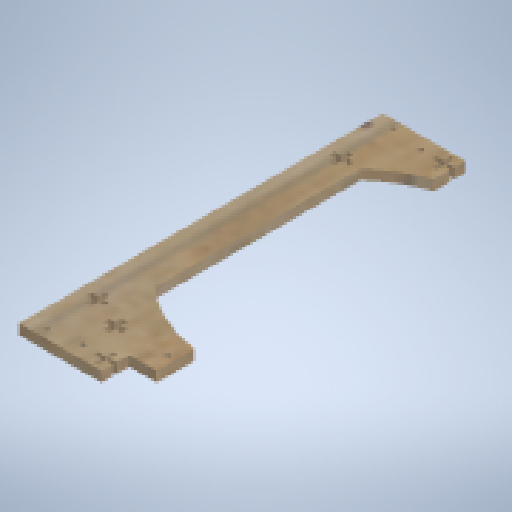
# Autodesk Inventor part: back_under
Saved by Autodesk Inventor 2024.1 (Build 281209000, 209)
## iProperties
Created: 2025-09-28
Part Number: back_under
Material: 木材 (カエデ材)
Document SubType Name: Modeling
Designer: hibik
Density: 0.67 g/cm^3
Appearance: ナチュラル カエデ材 - 光沢 濃い着色
Author: hibik
Autodesk Inventor part; units mm, degrees
ref_plane "YZ Plane" through (0, 0, 0) normal (1, 0, 0) x (0, 1, 0)
ref_plane "XZ Plane" through (0, 0, 0) normal (0, 1, 0) x (-1, 0, 0)
ref_plane "XY Plane" through (0, 0, 0) normal (0, 0, 1) x (1, 0, 0)
sketch "スケッチ1" plane through (0, 0, 0) normal (0, 1, 0) x (-1, 0, 0)
  line L0 (0, 99) -> (20, 99)
  line L1 (20, 99) -> (20, -99)
  line L2 (20, -99) -> (0, -99)
  line L3 (0, -99) -> (0, 99)
  point P0 (0, 0)
  point P1 (0, 0)
  dimension "d0" = 198
  dimension "d1" = 20
  constraints: 8 end point, 2 parallel, 1 coincident, 1 horizontal, 1 midpoint, 1 perpendicular
  measures "d0" distance of L0.end L1.end
  measures "d1" distance of L0.start L0.end
extrude "押し出し1" add sketch "スケッチ1" along normal blind 5.5
sketch "スケッチ2" plane through (0, 5.5, 0) normal (0, 1, 0) x (1, 0, 0)
  line L0 (-15, -67.8) -> (-5, -67.8)
  line L1 (-5, -67.8) -> (-5, -64.8)
  line L2 (-5, -64.8) -> (-15, -64.8)
  line L3 (-15, -64.8) -> (-15, -67.8)
  line L4 (-8.5, -71.3) -> (-11.5, -71.3)
  line L5 (-11.5, -71.3) -> (-11.5, -61.3)
  line L6 (-11.5, -61.3) -> (-8.5, -61.3)
  line L7 (-8.5, -61.3) -> (-8.5, -71.3)
  line L8 (-20, -99) -> (0, -99) projected
  circle A0 centre (-10, -94.3) radius 1.6
  point P0 (0, 0)
  point P1 (-8.5, -66.3)
  point P2 (-15, -66.3)
  point P3 (-10, -71.3)
  point P4 (-10, -67.8)
  point P5 (-10, -99)
  point P6 (-8.5, -64.8)
  point P7 (-11.5, -64.8)
  point P8 (-11.5, -67.8)
  point P9 (-8.5, -67.8)
  point P10 (-10, -99)
  dimension "d4" = 10
  dimension "d5" = 27.7
  dimension "d6" = 3
  dimension "d9" = 3.2
  dimension "d10" = 4.7
  constraints: 16 end point, 6 midpoint, 4 parallel, 4 perpendicular, 3 vertical alignment, 2 horizontal, 1 centre point, 1 horizontal alignment
  measures "d4" distance of L6.end L4.start
  measures "d5" distance between parallel lines of L8 L4
  measures "d6" distance of L4.start L4.end
  measures "d9" diameter of A0
  measures "d10" distance from line of L8 A0.centre
extrude "押し出し2" cut sketch "スケッチ2" against normal through all
sketch "スケッチ3" plane through (0, 5.5, 0) normal (0, 1, 0) x (1, 0, 0)
  line L0 (-172, 99) -> (-172, -99) projected
  line L1 (-172, -99) -> (-163.7059, -99) projected
  line L2 (25, -99) -> (25, -84) projected
  line L3 (25, -84) -> (40, -84) projected
  line L4 (40, -84) -> (40, -75.7059) projected
  line L5 (0, -44.9017) -> (0, 66.9017) projected
  line L6 (0, -99) -> (0, 99) projected
  line L7 (25, 99) -> (-8.2941, 99) projected
  arc A0 (0, -44.9017) -> (40, -63.3303) centre (50, 11) ccw projected
  arc A1 (25, 81.7107) -> (0, 66.9017) centre (50, 11) ccw projected
  line L8 (25, 81.7107) -> (25, 99) projected
  arc A2 (-160.2941, -99) -> (-163.7059, -99) centre (-162, -94.3) ccw projected
  line L9 (-160.2941, -99) -> (-11.7059, -99) projected
  arc A3 (-8.2941, -99) -> (-11.7059, -99) centre (-10, -94.3) ccw projected
  line L10 (-8.2941, -99) -> (25, -99) projected
  arc A4 (40, -72.2941) -> (40, -75.7059) centre (35.3, -74) ccw projected
  line L11 (40, -72.2941) -> (40, -63.3303) projected
  arc A5 (-11.7059, 99) -> (-8.2941, 99) centre (-10, 94.3) ccw projected
  line L12 (-11.7059, 99) -> (-160.2941, 99) projected
  arc A6 (-163.7059, 99) -> (-160.2941, 99) centre (-162, 94.3) ccw projected
  line L13 (-163.7059, 99) -> (-172, 99) projected
  circle A7 centre (7.35, -92) radius 5 projected
  circle A8 centre (7.35, 92) radius 5 projected
  line L14 (40, -72.2941) -> (40, -75.7059)
  point P0 (0, 0)
  point P1 (0, -19)
  point P2 (0, 66.9017)
  constraints: 2 end point, 1 vertical
extrude "押し出し3" add sketch "スケッチ3" against normal up to surface (5.5 mm away) contours L7 L8 A1 L6 | L6 A0 L11 A4 L4 L3 L2 L10 | L14 A4 | A7 | A8
sketch "スケッチ4" plane through (0, 5.5, 0) normal (0, 1, 0) x (1, 0, 0)
  line L0 (5.8, -79) -> (8.8, -79)
  line L1 (8.8, -79) -> (8.8, -69)
  line L2 (8.8, -69) -> (5.8, -69)
  line L3 (5.8, -69) -> (5.8, -79)
  line L4 (2.3, -75.5) -> (12.3, -75.5)
  line L5 (12.3, -75.5) -> (12.3, -72.5)
  line L6 (12.3, -72.5) -> (2.3, -72.5)
  line L7 (2.3, -72.5) -> (2.3, -75.5)
  line L8 (-11.5, -61.3) -> (-8.5, -61.3) projected
  line L9 (-8.5, -71.3) -> (-11.5, -71.3) projected
  line L10 (-5, -64.8) -> (-5, -67.8) projected
  line L11 (-20, 99) -> (-20, -99) projected
  line L12 (25, -84) -> (40, -84) projected
  line L13 (-20, -99) -> (25, -99) projected
  line L14 (40, -84) -> (40, -63.3303)
  circle A0 centre (35.3, -74) radius 1.6
  circle A1 centre (-10, -94.3) radius 1.6 projected
  point P0 (0, 0)
  point P1 (2.3, -74)
  point P2 (5.8, -74)
  point P3 (7.3, -79)
  point P4 (7.3, -75.5)
  point P5 (-10, -71.3)
  point P6 (12.3, -74)
  point P7 (5.8, -75.5)
  point P8 (8.8, -75.5)
  point P9 (8.8, -72.5)
  point P10 (5.8, -72.5)
  dimension "d13" = 10
  dimension "d14" = 10
  dimension "d15" = 10
  dimension "d16" = 10
  dimension "d17" = 27.7
  dimension "d18" = 27.7
  dimension "d21" = 4.7
  dimension "d22" = 4.7
  constraints: 18 end point, 6 midpoint, 4 parallel, 3 equal length, 2 horizontal, 2 horizontal alignment, 2 perpendicular, 1 centre point, 1 equal radius, 1 vertical alignment
  measures "d13" distance between parallel lines of L8 L9
  measures "d14" distance of L5.end L6.end
  measures "d15" distance from line of L11 point (-10, -71.3)
  measures "d16" distance from line of L12 point (12.3, -74)
  measures "d17" distance between parallel lines of L13 L9
  measures "d18" distance between parallel lines of L14 L5
  measures "d21" distance from line of L14 A0.centre
  measures "d22" distance from line of L13 A1.centre
extrude "押し出し4" cut sketch "スケッチ4" against normal through all contours L3 L4 L1 L0 | L4 L7 L6 L3 | L3 L6 L1 L4 | L1 L6 L5 L4 | L3 L2 L1 L6 | A0
mirror "ミラー1" about plane through (0, 0, 0) normal (0, 0, 1) of "押し出し2"
sketch "スケッチ5" plane through (0, 5.5, 0) normal (0, 1, 0) x (1, 0, 0)
  line L0 (25, -91) -> (15, -91)
  line L1 (15, -91) -> (15, -93)
  line L2 (15, -93) -> (25, -93)
  line L3 (25, -93) -> (25, -91)
  line L4 (19, -97) -> (21, -97)
  line L5 (21, -97) -> (21, -87)
  line L6 (21, -87) -> (19, -87)
  line L7 (19, -87) -> (19, -97)
  line L8 (25, -99) -> (25, -84) projected
  line L9 (-20, -99) -> (25, -99) projected
  circle A0 centre (7.35, -92) radius 1.6
  point P0 (0, 0)
  point P1 (25, -92)
  point P2 (15, -92)
  point P3 (19, -92)
  point P4 (20, -87)
  point P5 (20, -91)
  point P6 (19, -91)
  point P7 (19, -93)
  point P8 (21, -93)
  point P9 (21, -91)
  dimension "d25" = 10
  dimension "d26" = 7
  dimension "d27" = 2
  dimension "d28" = 3.2
  dimension "d29" = 17.65
  constraints: 16 end point, 5 midpoint, 4 parallel, 4 perpendicular, 2 horizontal, 2 horizontal alignment, 1 centre point, 1 collinear, 1 vertical alignment
  measures "d25" distance of L1.end L2.end
  measures "d26" distance from line of L9 point (25, -92)
  measures "d27" distance of L4.start L4.end
  measures "d28" diameter of A0
  measures "d29" distance from line of L8 A0.centre
extrude "押し出し5" cut sketch "スケッチ5" against normal through all
mirror "ミラー2" about plane through (0, 0, 0) normal (0, 0, 1) of "押し出し5"
equation "\"d14\" = d13"
equation "\"d16\" = d15"
equation "\"d18\" = d17"
equation "\"d21\" = d22"
